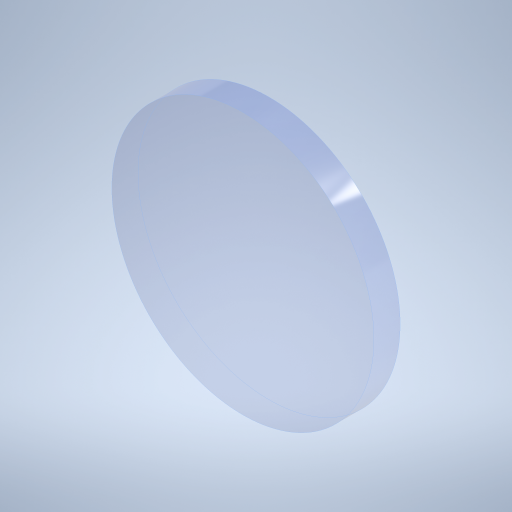
# Autodesk Inventor part: salt
Saved by Autodesk Inventor 2023 (Build 270158000, 158)
## iProperties
Created: 2023-01-24
Part Number: salt
Material: Water
Document SubType Name: Modeling
Designer: remidm
Density: 0.9983 g/cm^3
Appearance: Tropical Blue
Mass: 78.4063 g
Surface Area: 188.496 cm^2
Volume: 78.5398 cm^3
SaltDiameter: 80.000 mm
SaltThickness: 0.315 in
Author: remidm
Autodesk Inventor part; units mm, degrees
ref_plane "YZ Plane" through (0, 0, 0) normal (1, 0, 0) x (0, 1, 0)
ref_plane "XZ Plane" through (0, 0, 0) normal (0, 1, 0) x (-1, 0, 0)
ref_plane "XY Plane" through (0, 0, 0) normal (0, 0, 1) x (1, 0, 0)
sketch "Sketch1" plane through (0, 0, 0) normal (0, 0, 1) x (1, 0, 0)
  circle A0 centre (0, 0) radius 40
  dimension "SaltDiameter" = 80
  constraints: 1 centre point, 1 coincident
  measures "SaltDiameter" diameter of A0
extrude "Extrusion1" add sketch "Sketch1" along normal blind 8
body "Solid1"
